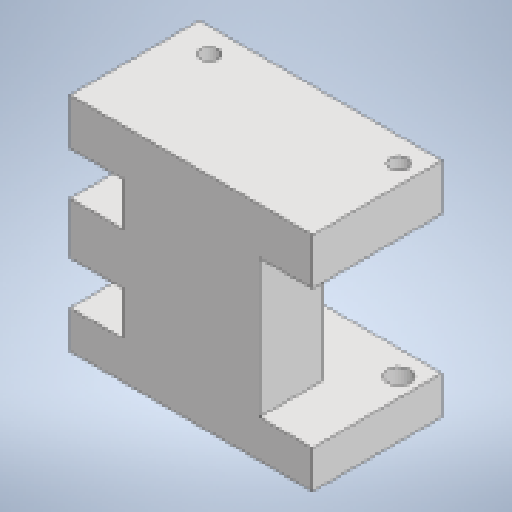
# Autodesk Inventor part: foot_bridge
Saved by Autodesk Inventor 2024 (Build 280153000, 153)
## iProperties
Created: 2024-09-17
Part Number: foot_bridge
Material: 일반
Document SubType Name: Modeling
Designer: Eungang
Density: 1 g/cm^3
Appearance: 기본값
Author: Eungang
Autodesk Inventor part; units mm, degrees
ref_plane "YZ Plane" through (0, 0, 0) normal (1, 0, 0) x (0, 1, 0)
ref_plane "XZ Plane" through (0, 0, 0) normal (0, 1, 0) x (-1, 0, 0)
ref_plane "XY Plane" through (0, 0, 0) normal (0, 0, 1) x (1, 0, 0)
sketch "스케치1" plane through (0, 0, 0) normal (0, 0, 1) x (1, 0, 0)
  line L0 (7.5, 38) -> (7.5, 36.5) projected
  line L1 (2, 38) -> (7.5, 38) projected
  line L2 (2, 38) -> (2, 8) projected
  line L3 (2, 8) -> (6.525, 8) projected
  line L4 (6.525, 10.5) -> (6.525, 8) projected
  line L5 (6.525, 10.5) -> (10.3997, 10.5) projected
  line L6 (10.3997, 10.5) -> (10.6003, 10.5) projected
  line L7 (10.6003, 10.5) -> (14.475, 10.5) projected
  line L8 (14.475, 10.5) -> (14.475, 8) projected
  line L9 (14.475, 8) -> (28.525, 8) projected
  line L10 (28.525, 10.5) -> (28.525, 8) projected
  line L11 (28.525, 10.5) -> (32.3997, 10.5) projected
  line L12 (32.3997, 10.5) -> (32.6003, 10.5) projected
  line L13 (32.6003, 10.5) -> (34.7876, 10.5) projected
  line L14 (34.7876, 10.5) -> (34.7876, 19.4) projected
  line L15 (36, 19.4) -> (34.7876, 19.4) projected
  line L16 (36, 24) -> (36, 19.4) projected
  line L17 (38.55, 24) -> (36, 24) projected
  line L18 (38.55, 24) -> (38.55, 25.4) projected
  line L19 (38.55, 25.4) -> (37.1, 25.4) projected
  line L20 (37.1, 25.4) -> (37.1, 35.5) projected
  line L21 (49.9, 35.5) -> (37.1, 35.5) projected
  line L22 (49.9, 25.4) -> (49.9, 35.5) projected
  line L23 (49.9, 25.4) -> (48.45, 25.4) projected
  line L24 (48.45, 24) -> (48.45, 25.4) projected
  line L25 (51, 24) -> (48.45, 24) projected
  line L26 (51, 24) -> (51, 10.5) projected
  line L27 (51, 10.5) -> (54.3997, 10.5) projected
  line L28 (54.3997, 10.5) -> (54.6003, 10.5) projected
  line L29 (54.6003, 10.5) -> (57.5, 10.5) projected
  line L30 (57.5, 36.5) -> (57.5, 10.5) projected
  line L31 (57.5, 36.5) -> (51.5, 36.5) projected
  line L32 (51.5, 38) -> (51.5, 36.5) projected
  line L33 (35.5, 38) -> (51.5, 38) projected
  line L34 (35.5, 36.5) -> (35.5, 38) projected
  line L35 (35.5, 36.5) -> (29.5, 36.5) projected
  line L36 (29.5, 38) -> (29.5, 36.5) projected
  line L37 (13.5, 38) -> (29.5, 38) projected
  line L38 (13.5, 36.5) -> (13.5, 38) projected
  line L39 (13.5, 36.5) -> (7.5, 36.5) projected
  line L40 (22.05, 14.2) -> (27.95, 14.2) projected
  line L41 (22.05, 18) -> (22.05, 14.2) projected
  line L42 (27.95, 18) -> (22.05, 18) projected
  line L43 (27.95, 14.2) -> (27.95, 18) projected
  line L44 (34.6876, 10.6) -> (7.6, 10.6)
  line L45 (7.6, 10.6) -> (7.6, 36.4)
  line L46 (7.6, 36.4) -> (34.6876, 36.4)
  line L47 (34.6876, 36.4) -> (34.6876, 10.6)
  line L48 (7.6, 36.4) -> (6.525, 36.4)
  line L49 (7.6, 10.6) -> (6.525, 10.6)
  line L50 (6.525, 10.6) -> (6.525, 36.4)
  line L51 (6.525, 36.4) -> (7.6, 36.4)
  line L52 (7.6, 36.4) -> (7.6, 10.6)
  point P0 (0, 0)
  constraints: 18 end point, 4 parallel, 2 perpendicular, 1 horizontal
extrude "돌출1" add sketch "스케치1" along normal blind 15 contours L41 L42 L43 L40 | L44 L45 L46 L47 | L49 L50 L48 L45
sketch "스케치2" plane through (0, 0, 15) normal (0, 0, 1) x (1, 0, 0)
  line L0 (34.5, 38) -> (52.5, 38) projected
  line L1 (52.5, 38) -> (52.5, 36.5) projected
  line L2 (56.5, 36.5) -> (52.5, 36.5) projected
  line L3 (56.5, 38) -> (56.5, 36.5) projected
  line L4 (56.5, 38) -> (59.1, 38) projected
  line L5 (59.1, 38) -> (59.1, 40) projected
  line L6 (6, 40) -> (59.1, 40) projected
  line L7 (6, 38) -> (6, 40) projected
  line L8 (6, 38) -> (8.5, 38) projected
  line L9 (8.5, 38) -> (8.5, 36.5) projected
  line L10 (12.5, 36.5) -> (8.5, 36.5) projected
  line L11 (12.5, 38) -> (12.5, 36.5) projected
  line L12 (12.5, 38) -> (30.5, 38) projected
  line L13 (30.5, 38) -> (30.5, 36.5) projected
  line L14 (34.5, 36.5) -> (30.5, 36.5) projected
  line L15 (34.5, 38) -> (34.5, 36.5) projected
  line L16 (14.475, 10.5) -> (12.975, 10.5) projected
  line L17 (12.975, 10.5) -> (12.975, 8.5) projected
  line L18 (12.975, 8.5) -> (8.025, 8.5) projected
  line L19 (8.025, 10.5) -> (8.025, 8.5) projected
  line L20 (8.025, 10.5) -> (6.525, 10.5) projected
  line L21 (6.525, 10.5) -> (6.525, 8) projected
  line L22 (6, 8) -> (6.525, 8) projected
  line L23 (6, 8) -> (6, 6) projected
  line L24 (6, 6) -> (59.1, 6) projected
  line L25 (59.1, 8) -> (59.1, 6) projected
  line L26 (58.475, 8) -> (59.1, 8) projected
  line L27 (58.475, 8) -> (58.475, 10.5) projected
  line L28 (58.475, 10.5) -> (56.975, 10.5) projected
  line L29 (56.975, 10.5) -> (56.975, 8.5) projected
  line L30 (56.975, 8.5) -> (52.025, 8.5) projected
  line L31 (52.025, 10.5) -> (52.025, 8.5) projected
  line L32 (52.025, 10.5) -> (50.525, 10.5) projected
  line L33 (50.525, 10.5) -> (50.525, 8) projected
  line L34 (36.475, 8) -> (50.525, 8) projected
  line L35 (36.475, 8) -> (36.475, 10.5) projected
  line L36 (36.475, 10.5) -> (34.975, 10.5) projected
  line L37 (34.975, 10.5) -> (34.975, 8.5) projected
  line L38 (34.975, 8.5) -> (30.025, 8.5) projected
  line L39 (30.025, 10.5) -> (30.025, 8.5) projected
  line L40 (30.025, 10.5) -> (28.525, 10.5) projected
  line L41 (28.525, 10.5) -> (28.525, 8) projected
  line L42 (14.475, 8) -> (28.525, 8) projected
  line L43 (14.475, 8) -> (14.475, 10.5) projected
  line L44 (14.475, 36.4) -> (28.525, 36.4)
  line L45 (34.6876, 10.6) -> (34.6876, 36.4) projected
  line L46 (14.475, 10.6) -> (28.525, 10.6)
  line L47 (28.525, 10.6) -> (28.525, 36.4)
  line L48 (28.525, 36.4) -> (14.475, 36.4)
  line L49 (-13.0231, 23) -> (78.1205, 23)
  line L50 (14.5, -11.1) -> (14.5, 56.1)
  line L51 (34.6876, 36.4) -> (6.525, 36.4) projected
  line L52 (6.525, 36.4) -> (6.525, 10.6) projected
  line L53 (6.525, 10.6) -> (34.6876, 10.6) projected
  line L54 (28.525, 23) -> (34.6876, 23)
  line L55 (34.6876, 23) -> (34.6876, 31)
  line L56 (34.6876, 31) -> (28.525, 31)
  line L57 (28.525, 31) -> (28.525, 23)
  line L58 (28.525, 23) -> (34.6876, 23)
  line L59 (34.6876, 23) -> (34.6876, 15)
  line L60 (34.6876, 15) -> (28.525, 15)
  line L61 (28.525, 15) -> (28.525, 23)
  line L62 (6.525, 23) -> (12.688, 23)
  line L63 (12.688, 23) -> (12.688, 31)
  line L64 (12.688, 31) -> (6.525, 31)
  line L65 (6.525, 31) -> (6.525, 23)
  line L66 (14.5, 57.1) -> (14.5, -10.1)
  line L67 (12.688, 23) -> (12.688, 15)
  line L68 (12.688, 15) -> (6.525, 15)
  line L69 (6.525, 15) -> (6.525, 23)
  line L70 (6.525, 36.4) -> (6.525, 10.6) projected
  line L71 (12.688, 23) -> (6.525, 23)
  line L72 (6.525, 23) -> (6.525, 26)
  line L73 (6.525, 26) -> (12.688, 26)
  line L74 (12.688, 26) -> (12.688, 23)
  line L75 (12.688, 23) -> (6.525, 23)
  line L76 (6.525, 23) -> (6.525, 20)
  line L77 (6.525, 20) -> (12.688, 20)
  line L78 (12.688, 20) -> (12.688, 23)
  point P0 (0, 0)
  dimension "d3" = 6.163
  dimension "d4" = 8
  constraints: 60 end point, 11 parallel, 8 point on line, 7 horizontal, 6 perpendicular, 4 symmetric about line, 1 vertical, 4 other
  measures "d3" distance of L64.end L63.end
  measures "d4" distance of L63.end L62.end
extrude "돌출2" cut sketch "스케치2" against normal up to next contours L64 L63 L73 L52 | L56 L45 L49 L47 | L49 L45 L60 L47 | L67 L68 L52 L77
sketch "스케치4" plane through (6.525, 10.6, 0) normal (0, -1, 0) x (1, 0, 0)
  circle A0 centre (3.975, 2.8) radius 1.35 projected
  circle A1 centre (25.975, 2.8) radius 1.35
  circle A2 centre (25.975, 2.8) radius 1.55
  circle A3 centre (3.975, 2.8) radius 1.55
  point P0 (-6.525, 0)
  dimension "d14" = 0.2
  dimension "d15" = 0.2
  constraints: 3 centre point
  measures "d14" radial gap between concentric circles of A1 A2
  measures "d15" radial gap between concentric circles of A0 A3
extrude "돌출4" cut sketch "스케치4" against normal up to next contours A0 | A1
sketch "스케치5" plane through (6.525, 36.4, 0) normal (0, 1, 0) x (1, 0, 0)
  circle A0 centre (25.975, -2.8) radius 1.025 projected
  circle A1 centre (3.975, -2.8) radius 1.025 projected
  circle A2 centre (25.975, -2.8) radius 1.225
  circle A3 centre (3.975, -2.8) radius 1.225
  point P0 (-6.525, 0)
  dimension "d16" = 0.2
  dimension "d17" = 0.2
  constraints: 2 centre point
  measures "d16" radial gap between concentric circles of A0 A2
  measures "d17" radial gap between concentric circles of A1 A3
extrude "돌출5" cut sketch "스케치5" against normal up to next contours A0 | A1
sketch "스케치6" plane through (0, 0, 0) normal (0, 0, -1) x (-1, 0, 0)
  line L0 (-28.525, 31) -> (-34.6876, 31) projected
  line L1 (-34.6876, 31) -> (-34.6876, 36.4) projected
  line L2 (-34.6876, 36.4) -> (-6.525, 36.4) projected
  line L3 (-6.525, 36.4) -> (-6.525, 31) projected
  line L4 (-6.525, 31) -> (-12.688, 31) projected
  line L5 (-12.688, 31) -> (-12.688, 26) projected
  line L6 (-12.688, 26) -> (-6.525, 26) projected
  line L7 (-6.525, 26) -> (-6.525, 20) projected
  line L8 (-6.525, 20) -> (-12.688, 20) projected
  line L9 (-12.688, 20) -> (-12.688, 15) projected
  line L10 (-12.688, 15) -> (-6.525, 15) projected
  line L11 (-6.525, 15) -> (-6.525, 10.6) projected
  line L12 (-6.525, 10.6) -> (-34.6876, 10.6) projected
  line L13 (-34.6876, 10.6) -> (-34.6876, 15) projected
  line L14 (-34.6876, 15) -> (-28.525, 15) projected
  line L15 (-28.525, 15) -> (-28.525, 31) projected
  line L16 (-12.688, 31) -> (-28.525, 31)
  line L17 (-28.525, 31) -> (-28.525, 15)
  line L18 (-28.525, 15) -> (-12.688, 15)
  line L19 (-12.688, 15) -> (-12.688, 31)
  line L20 (13.0231, 24) -> (-78.1205, 24)
  line L21 (-14.5, 58.1) -> (-14.5, -9.1)
  point P0 (0, 0)
  constraints: 12 end point, 2 horizontal, 2 parallel, 1 perpendicular, 1 vertical, 4 other
extrude "돌출6" cut sketch "스케치6" against normal blind 7.5 contours L16 L21 L20 L15 | L20 L21 L18 L15 | L16 L5 L19 L20 L21 | L20 L19 L9 L18 L21 | L20 L7 L8 L19 | L19 L6 L7 L20
sketch "스케치7" plane through (0, 0, 15) normal (0, 0, 1) x (1, 0, 0)
  circle A0 centre (14.5, 24) radius 1.55 projected
  point P0 (0, 0)
extrude "돌출7" cut sketch "스케치7" against normal up to next
